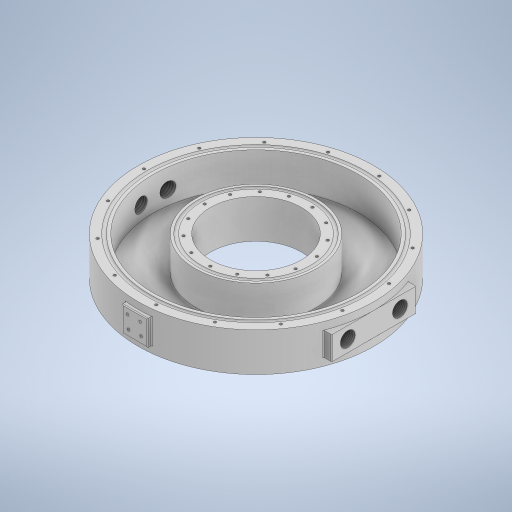
# Autodesk Inventor part: BioCoilCad_v3
Saved by Autodesk Inventor 2023 (Build 270158000, 158)
## iProperties
Created: 2023-02-06
Part Number: BioCoilCad_v3
Material: Generic
Document SubType Name: Modeling
Designer: QuBiT Data PC
Density: 1 g/cm^3
Appearance: Default
Author: QuBiT Data PC
Autodesk Inventor part; units mm, degrees
ref_plane "XZ Plane" through (0, 0, 0) normal (0, 1, 0) x (-1, 0, 0)
sketch "Sketch1" plane through (0, 0, 0) normal (1, 0, 0) x (0, 1, 0)
  line L0 (0.0002, -27) -> (0.0002, -70)
  line L1 (0.0002, -70) -> (23.0002, -70)
  line L2 (23.0002, -61) -> (3.0002, -61)
  line L3 (3.0002, -61) -> (3.0002, -36)
  line L4 (3.0002, -36) -> (23.0002, -36)
  line L5 (23.0002, -27) -> (0.0002, -27)
  line L6 (30.1625, 0) -> (-33.3375, 0)
  arc A0 (23.0002, -32.5) -> (23.0002, -34.5) centre (23.0002, -33.5) ccw
  arc A1 (23.0002, -62.8) -> (23.0002, -64.8) centre (23.0002, -63.8) ccw
  line L7 (23.0002, -27) -> (23.0002, -32.5)
  line L8 (23.0002, -34.5) -> (23.0002, -36)
  line L9 (23.0002, -61) -> (23.0002, -62.8)
  line L10 (23.0002, -64.8) -> (23.0002, -70)
  point P0 (0, 0)
  dimension "d3" = 27
  dimension "d52" = 3
  dimension "d76" = 20
  dimension "d77" = 20
  dimension "d78" = 33.5
  dimension "d79" = 63.8
  dimension "d80" = 9
  dimension "d81" = 9
  dimension "d152" = 70
  dimension "d153" = 1
  dimension "d154" = 1
  constraints: 22 end point, 5 vertical, 4 perpendicular, 4 point on circle, 2 centre point, 2 coincident, 1 horizontal
  measures "d3" distance from line of point (0, 0) L5
  measures "d52" distance between parallel lines of L0 L3
  measures "d76" distance of L3.end L4.end
  measures "d77" distance of L2.start L2.end
  measures "d78" vertical distance of point (23, -33.5) point (0, 0)
  measures "d79" vertical distance of point (23, -63.8) point (0, 0)
  measures "d80" distance of L5.start L4.end
  measures "d81" distance of L2.start L1.end
  measures "d152" distance between parallel lines of L1 L6
  measures "d153" radius of A0
  measures "d154" radius of A1
revolve "Revolution1" add sketch "Sketch1" angle 360 about axis through (0, 30.1625, 0) along (0, -1, 0)
sketch "Sketch8" plane through (0, 23.0002, 0) normal (0, 1, 0) x (1, 0, 0)
  point P0 (0, 0)
  point P1 (-66.6, 0)
  point P2 (-30.5, 0)
  dimension "d84" = 30.5
  dimension "d85" = 66.6
  measures "d84" distance of point (0, 0) point (-30.5, 0)
  measures "d85" distance of point (0, 0) point (-66.6, 0)
hole "Hole7" at (-66.6, 23.0002, 0) at (-30.5, 23.0002, 0) direction (0, -1, 0) diameter 1.567 depth 6.3 thread size "M2x0.4" class "6H" standard "ISO Metric profile"
pattern_circular "Circular Pattern7" count 15 over 360 about axis through (0, 11.5002, 0) along (0, -1, 0) of "Hole7"
ref_plane "Work Plane1" through (0, 11.5002, 70) normal (0, 0, 1) x (1, 0, 0)
ref_plane "Work Plane2" through (0, 11.5002, -70) normal (0, 0, 1) x (1, 0, 0)
sketch "Sketch15" plane through (0, 0.0002, 0) normal (0, -1, 0) x (1, 0, 0)
  point P0 (0, 0)
ref_plane "Work Plane4" through (70, 11.5002, 0) normal (1, 0, 0) x (0, 1, 0)
sketch "Sketch18" plane through (70, 11.5002, 0) normal (1, 0, 0) x (0, 1, 0)
  line L0 (7, -25) -> (-7, -25)
  line L1 (-7, -25) -> (-7, 25)
  line L2 (-7, 25) -> (7, 25)
  line L3 (7, 25) -> (7, -25)
  point P0 (-11.5002, 0)
  dimension "d131" = 50
  dimension "d132" = 14
  constraints: 8 end point, 2 parallel, 1 horizontal, 1 perpendicular
  measures "d131" distance between parallel lines of L2 L0
  measures "d132" distance between parallel lines of L1 L3
extrude "Extrusion4" add sketch "Sketch18" against normal blind 6
fillet "Fillet3" radius 0.5 2 edges at (70, 11.5002, -25) (70, 11.5002, 25)
sketch "Sketch21" plane through (0, 0.0002, 0) normal (0, -1, 0) x (1, 0, 0)
  point P0 (0, 0)
ref_plane "Work Plane5" through (0, 11.5002, 70) normal (0, 0, 1) x (1, 0, 0)
sketch "Sketch22" plane through (0, 11.5002, 70) normal (0, 0, 1) x (1, 0, 0)
  line L0 (-7.5, 7.5) -> (7.5, 7.5)
  line L1 (7.5, 7.5) -> (7.5, -7.5)
  line L2 (7.5, -7.5) -> (-7.5, -7.5)
  line L3 (-7.5, -7.5) -> (-7.5, 7.5)
  point P0 (0, -11.5002)
  dimension "d155" = 15
  dimension "d156" = 15
  constraints: 8 end point, 2 parallel, 1 horizontal, 1 perpendicular
  measures "d155" distance of L0.start L0.end
  measures "d156" distance of L2.end L0.start
extrude "Extrusion6" add sketch "Sketch22" along normal blind 2 and the other way blind 2
sketch "Sketch23" plane through (0, 11.5002, 72) normal (0, 0, 1) x (1, 0, 0)
  line L0 (-70, 11.5) -> (70, 11.5) projected
  line L1 (7.5, 7.5) -> (-7.5, 7.5) projected
  line L2 (7.5, -7.5) -> (7.5, 7.5) projected
  point P0 (0, -11.5002)
  point P1 (3.175, 3.75)
  point P2 (-4.325, 3.75)
  point P3 (-3.75, -3.75)
  point P4 (3.75, -3.4094)
  dimension "d163" = 7.5
  dimension "d164" = 7.5
  dimension "d165" = 7.5
  dimension "d166" = 3.75
  dimension "d167" = 3.75
  dimension "d168" = 3.75
  measures "d163" distance of point (3.175, 3.75) point (-4.325, 3.75)
  measures "d164" vertical distance of point (-3.75, -3.75) point (-4.325, 3.75)
  measures "d165" horizontal distance of point (3.75, -3.409) point (-3.75, -3.75)
  measures "d166" distance from line of L1 point (3.175, 3.75)
  measures "d167" distance from line of L1 point (-4.325, 3.75)
  measures "d168" distance from line of L2 point (3.75, -3.409)
hole "Hole11" at (-4.325, 15.2502, 72) at (-3.75, 7.7502, 72) at (3.75, 8.0909, 72) at (3.175, 15.2502, 72) direction (0, 0, -1) diameter 1.567 depth 8 thread size "M2x0.4" class "6H" standard "ISO Metric profile"
ref_plane "Work Plane6" through (0, 11.5002, -70) normal (0, 0, 1) x (1, 0, 0)
sketch "Sketch24" plane through (0, 11.5002, -70) normal (0, 0, 1) x (1, 0, 0)
  line L0 (7.5, 7.5) -> (-7.5, 7.5)
  line L1 (-7.5, 7.5) -> (-7.5, -7.5)
  line L2 (-7.5, -7.5) -> (7.5, -7.5)
  line L3 (7.5, -7.5) -> (7.5, 7.5)
  point P0 (0, -11.5002)
  point P1 (-3.175, 3.75)
  point P2 (4.325, 3.75)
  point P3 (3.75, -3.75)
  point P4 (-3.75, -3.75)
  dimension "d176" = 15
  dimension "d177" = 15
  dimension "d178" = 3.75
  dimension "d179" = 3.75
  dimension "d180" = 3.75
  dimension "d181" = 3.75
  dimension "d182" = 7.5
  dimension "d183" = 7.5
  constraints: 8 end point, 2 parallel, 1 horizontal, 1 perpendicular
  measures "d176" distance of L0.start L0.end
  measures "d177" distance of L2.end L0.start
  measures "d178" distance from line of L0 point (-3.175, 3.75)
  measures "d179" distance from line of L0 point (4.325, 3.75)
  measures "d180" distance from line of L2 point (3.75, -3.75)
  measures "d181" distance from line of L2 point (-3.75, -3.75)
  measures "d182" distance of point (-3.175, 3.75) point (4.325, 3.75)
  measures "d183" distance of point (-3.75, -3.75) point (3.75, -3.75)
extrude "Extrusion7" add sketch "Sketch24" along normal blind 2 and the other way blind 2
sketch "Sketch25" plane through (0, 11.5002, -72) normal (0, 0, -1) x (-1, 0, 0)
  line L0 (7.5, 7.5) -> (-7.5, 7.5) projected
  line L1 (7.5, -7.5) -> (7.5, 7.5) projected
  line L2 (-7.5, -7.5) -> (7.5, -7.5) projected
  line L3 (-7.5, 7.5) -> (-7.5, -7.5) projected
  point P0 (0, -11.5002)
  point P1 (-3.75, -3.75)
  point P2 (-3.75, 3.75)
  point P3 (3.75, 3.75)
  point P4 (3.75, -3.75)
  dimension "d188" = 7.5
  dimension "d189" = 7.5
  dimension "d190" = 7.5
  dimension "d191" = 7.5
  dimension "d192" = 3.75
  dimension "d193" = 3.75
  dimension "d194" = 3.75
  dimension "d195" = 3.75
  measures "d188" distance of point (-3.75, 3.75) point (-3.75, -3.75)
  measures "d189" distance of point (3.75, 3.75) point (3.75, -3.75)
  measures "d190" distance of point (-3.75, 3.75) point (3.75, 3.75)
  measures "d191" distance of point (-3.75, -3.75) point (3.75, -3.75)
  measures "d192" distance from line of L0 point (3.75, 3.75)
  measures "d193" distance from line of L1 point (3.75, -3.75)
  measures "d194" distance from line of L2 point (-3.75, -3.75)
  measures "d195" distance from line of L3 point (-3.75, 3.75)
hole "Hole12" at (3.75, 15.2502, -72) at (-3.75, 15.2502, -72) at (-3.75, 7.7502, -72) at (3.75, 7.7502, -72) direction (0, 0, 1) diameter 1.567 depth 8 thread size "M2x0.4" class "6H" standard "ISO Metric profile"
fillet "Fillet4" radius 0.5 8 edges at (-7.5, 11.5002, -72) (0, 19.0002, -72) (7.5, 11.5002, -72) (0, 4.0002, -72) (7.5, 11.5002, 72) (0, 19.0002, 72) (-7.5, 11.5002, 72) (0, 4.0002, 72)
fillet "Fillet5" radius 0.8 1 edges at (65.3835, 11.5002, -25)
fillet "Fillet6" radius 0.8 5 edges at (65.3835, 11.5002, 25) (7.5, 11.5002, 69.5971) (-7.5, 11.5002, 69.5971) (-7.5, 11.5002, -69.5971) (7.5, 11.5002, -69.5971)
sketch "Sketch26" plane through (70, 11.5002, 0) normal (1, 0, 0) x (0, 0, -1)
  line L0 (25.5085, -7) -> (25.5085, 7) projected
  line L1 (-25.5085, 7) -> (-25.5085, -7) projected
  point P0 (0, -11.5002)
  point P1 (15.5085, 0)
  point P2 (-15.5085, 0)
  dimension "d206" = 10
  dimension "d207" = 10
  measures "d206" distance from line of L0 point (15.508, 0)
  measures "d207" distance from line of point (-15.508, 0) L1
hole "Hole13" at (70, 11.5002, 15.5085) at (70, 11.5002, -15.5085) direction (-1, 0, 0) diameter 7.9502 depth 14 taper from width 8.7371 to width 8.3632 over 5.9842 thread size "1/8" designation "1/8 - 27 NPT" standard "NPT for PVC Pipe and Fitting"
thread "Thread1" size "M2x0.4" class "6H" standard "ANSI Metric M Profile" full length
thread "Thread2" size "M2x0.4" class "6H" standard "ANSI Metric M Profile" full length
thread "Thread3" size "M2x0.4" class "6H" standard "ANSI Metric M Profile" full length
thread "Thread4" size "M2x0.4" class "6H" standard "ANSI Metric M Profile" full length
thread "Thread5" size "M2x0.4" class "6H" standard "ANSI Metric M Profile" full length
thread "Thread6" size "M2x0.4" class "6H" standard "ANSI Metric M Profile" full length
thread "Thread7" size "M2x0.4" class "6H" standard "ANSI Metric M Profile" full length
thread "Thread8" size "M2x0.4" class "6H" standard "ANSI Metric M Profile" full length
thread "Thread9" size "M2x0.4" class "6H" standard "ANSI Metric M Profile" full length
thread "Thread10" size "M2x0.4" class "6H" standard "ANSI Metric M Profile" full length
sketch "Sketch27" plane through (0, 0, 0) normal (1, 0, 0) x (0, 1, 0)
  point P0 (0, 0)
sketch "Sketch28" plane through (0, 0, 0) normal (1, 0, 0) x (0, 1, 0)
  point P0 (0, 0)
sketch "Sketch29" plane through (0, 0, 0) normal (1, 0, 0) x (0, 1, 0)
  point P0 (0, 0)
sketch "Sketch30" plane through (0, 0, 0) normal (1, 0, 0) x (0, 1, 0)
  point P0 (0, 0)
sketch "Sketch31" plane through (0, 0, 0) normal (1, 0, 0) x (0, 1, 0)
  point P0 (0, 0)
ref_plane "Work Plane7" through (-70, 11.5002, 0) normal (1, 0, 0) x (0, 1, 0)
sketch "Sketch32" plane through (-70, 11.5002, 0) normal (1, 0, 0) x (0, 1, 0)
  line L0 (5, -15) -> (-5, -15)
  line L1 (-5, -15) -> (-5, 15)
  line L2 (-5, 15) -> (5, 15)
  line L3 (5, 15) -> (5, -15)
  point P0 (-11.5002, 0)
  point P1 (0, 8)
  point P2 (0, -8)
  dimension "d237" = 30
  dimension "d238" = 10
  dimension "d240" = 7
  dimension "d241" = 7
  constraints: 8 end point, 2 parallel, 1 horizontal, 1 perpendicular
  measures "d237" distance of L2.end L0.start
  measures "d238" distance of L0.start L0.end
  measures "d240" distance from line of L2 point (0, 8)
  measures "d241" distance from line of L0 point (0, -8)
extrude "Extrusion8" add sketch "Sketch32" along normal blind 4
fillet "Fillet7" radius 1 4 edges at (-70, 11.5002, -15) (-70, 11.5002, 15) (-68.374, 11.5002, -15) (-68.374, 11.5002, 15)
sketch "Sketch33" plane through (-70, 11.5002, 0) normal (-1, 0, 0) x (0, 0, 1)
  line L0 (15.767, -5) -> (15.767, 5) projected
  line L1 (-14.9961, -5) -> (-14.9961, 5) projected
  line L2 (14.9961, 5) -> (14.9961, -5) projected
  point P0 (0, -11.5002)
  point P1 (7.9961, 0)
  point P2 (-7.9961, 0)
  point P3 (15.767, 0)
  point P4 (7.9961, 0)
  dimension "d246" = 7
  dimension "d247" = 7
  constraints: 1 coincident, 1 midpoint
  measures "d246" distance from line of L1 point (-7.996, 0)
  measures "d247" distance from line of L2 point (7.996, 0)
hole "Hole14" at (-70, 11.5002, -7.9961) at (-70, 11.5002, 7.9961) direction (1, 0, 0) diameter 8.376 depth 27.3 tip angle 118 thread size "M10x1.5" class "6H" standard "ANSI Metric M Profile"
body "Solid1"
